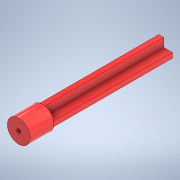
# Autodesk Inventor part: Bistable Rod 2
Saved by Autodesk Inventor 2020 (Build 240168000, 168)
## iProperties
Created: 2019-11-20
Part Number: Bistable Rod 2
Material: Generic
Document SubType Name: Modeling
Designer: camde
Density: 1 g/cm^3
Appearance: Light Red
Mass: 79.7328 g
Surface Area: 217.3 cm^2
Volume: 79.7328 cm^3
Author: camde
Autodesk Inventor part; units mm, degrees
ref_plane "YZ Plane" through (0, 0, 0) normal (1, 0, 0) x (0, 1, 0)
ref_plane "XZ Plane" through (0, 0, 0) normal (0, 1, 0) x (-1, 0, 0)
ref_plane "XY Plane" through (0, 0, 0) normal (0, 0, 1) x (1, 0, 0)
sketch "Sketch1" plane through (0, 0, 0) normal (0, 0, 1) x (1, 0, 0)
  line L0 (-4.7594, 8.1062) -> (1.01, 8.1062)
  line L1 (1.01, 8.1062) -> (1.01, -1.7998)
  line L2 (1.01, -1.7998) -> (10.916, -1.7998)
  line L3 (10.916, -1.7998) -> (10.916, -7.5692)
  line L4 (10.916, -4.6845) -> (-5.4983, -4.6845) construction
  line L5 (-1.8747, 8.1062) -> (-1.8747, -4.6845) construction
  line L6 (-14.6654, -7.5692) -> (-14.6654, -1.7998)
  line L7 (-14.6654, -1.7998) -> (-4.7594, -1.7998)
  line L8 (-4.7594, -1.7998) -> (-4.7594, 8.1062)
  line L9 (1.01, -17.4752) -> (-4.7594, -17.4752)
  line L10 (-4.7594, -17.4752) -> (-4.7594, -7.5692)
  line L11 (-4.7594, -7.5692) -> (-14.6654, -7.5692)
  line L12 (10.916, -1.7998) -> (10.916, -7.5692)
  line L13 (10.916, -7.5692) -> (1.01, -7.5692)
  line L14 (1.01, -7.5692) -> (1.01, -17.4752)
  point P0 (0, 0)
  point P1 (-14.6654, -4.6845)
  point P2 (-1.8747, -17.4752)
  point P3 (10.916, -4.6845)
  dimension "d0" = 5.7694
  dimension "d1" = 9.906
  dimension "d2" = 9.906
  dimension "d3" = 5.7694
  dimension "d6" = 360
  constraints: 30 end point, 3 perpendicular, 2 horizontal, 2 midpoint, 1 coincident, 1 point on line, 1 vertical, 33 other
  measures "d0" distance of L0.start L0.end
  measures "d1" distance of L0.end L1.end
  measures "d2" distance of L1.end L2.end
  measures "d3" distance of L2.end L3.end
extrude "Extrusion1" add sketch "Sketch1" along normal blind 108.8571
sketch "Sketch2" plane through (0, 0, 108.8571) normal (0, 0, 1) x (1, 0, 0)
  line L0 (-14.6654, -1.7998) -> (-14.6654, -7.5692) projected
  line L1 (-14.6654, -4.6845) -> (0, -4.6845) construction
  line L2 (1.01, 8.1062) -> (-4.7594, 8.1062) projected
  circle A0 centre (-1.8747, -4.6845) radius 13.112
  point P0 (0, 0)
  constraints: 2 end point, 1 horizontal, 1 midpoint, 1 point on line, 3 other
extrude "Extrusion2" add sketch "Sketch2" along normal blind 27.2143
sketch "Sketch3" plane through (0, 0, 0) normal (0, 0, -1) x (-1, 0, 0)
  line L0 (4.7594, -1.7998) -> (14.6654, -1.7998) projected
  line L1 (-1.01, -7.5692) -> (-10.916, -7.5692) projected
  line L2 (-10.916, -1.7998) -> (-10.916, -7.5692)
  line L3 (14.6654, -7.5692) -> (14.6654, -1.7998)
  line L4 (-1.01, -1.7998) -> (-1.01, 8.1062) projected
  circle A0 centre (1.8747, -4.6845) radius 13.112 construction
  line L5 (-1.01, 8.1062) -> (4.7594, 8.1062)
  line L6 (4.7594, -17.4752) -> (-1.01, -17.4752)
  line L7 (4.7594, 8.1062) -> (4.7594, -1.7998)
  line L8 (4.7594, -7.5692) -> (4.7594, -17.4752)
  line L9 (14.6654, -1.7998) -> (4.7594, -1.7998)
  line L10 (-1.01, -1.7998) -> (-10.916, -1.7998)
  line L11 (-1.01, -17.4752) -> (-1.01, -7.5692)
  line L12 (-1.01, -1.7998) -> (-1.01, 8.1062)
  line L13 (-10.916, -7.5692) -> (-1.01, -7.5692)
  line L14 (4.7594, -7.5692) -> (14.6654, -7.5692)
  point P0 (0, 0)
  constraints: 24 end point, 10 parallel, 4 perpendicular, 3 horizontal, 1 point on circle
extrude "Extrusion3" add sketch "Sketch3" along normal blind 27.2143
sketch "Sketch4" plane through (-1.8747, -4.6845, 136.0714) normal (0, 0, 1) x (1, 0, 0)
  circle A0 centre (0, 0) radius 2.3
  point P0 (1.8747, 4.6845)
  dimension "d14" = 4.6
  constraints: 1 centre point
  measures "d14" diameter of A0
extrude "Extrusion4" cut sketch "Sketch4" against normal blind 3.2
body "Solid1"
